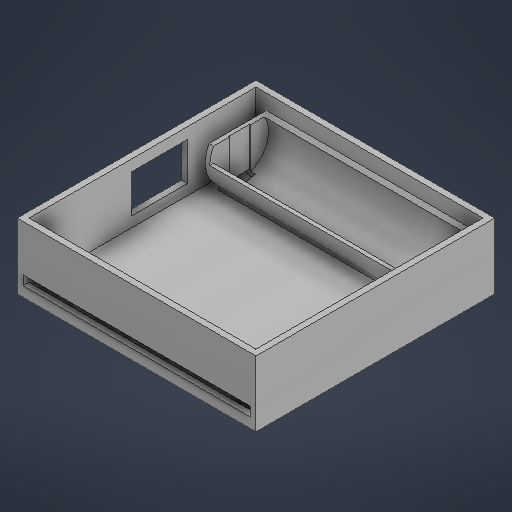
# Autodesk Inventor part: obudowa2
Saved by Autodesk Inventor 2026.1 (Build 301233000, 233)
## iProperties
Created: 2025-08-19
Part Number: obudowa2
Material: Generic
Document SubType Name: Modeling
Designer: Paweł
Density: 1 g/cm^3
Appearance: Light Gray
Mass: 30.7875 g
Surface Area: 279.129 cm^2
Volume: 30.7875 cm^3
Author: Paweł
Autodesk Inventor part; units mm, degrees
ref_plane "YZ Plane" through (0, 0, 0) normal (1, 0, 0) x (0, 1, 0)
ref_plane "XZ Plane" through (0, 0, 0) normal (0, 1, 0) x (-1, 0, 0)
sketch "Sketch1" plane through (0, 0, 0) normal (0, 1, 0) x (-1, 0, 0)
  line L0 (77.0121, 67.7143) -> (-2.9879, 67.7143)
  line L1 (-2.9879, 67.7143) -> (-2.9879, -12.2857)
  line L2 (-2.9879, -12.2857) -> (77.0121, -12.2857)
  line L3 (77.0121, -12.2857) -> (77.0121, 67.7143)
  point P0 (0, 0)
  dimension "d0" = 80
  dimension "d1" = 80
  constraints: 8 end point, 2 parallel, 1 horizontal, 1 perpendicular
  measures "d0" distance of L2.end L1.end
  measures "d1" distance of L0.end L1.end
extrude "Extrusion1" add sketch "Sketch1" along normal blind 2
sketch "Sketch2" plane through (0, 2, 0) normal (0, 1, 0) x (1, 0, 0)
  line L0 (2.9879, -67.7143) -> (2.9879, 12.2857) projected
  line L1 (2.9879, 12.2857) -> (-77.0121, 12.2857) projected
  line L2 (-77.0121, 12.2857) -> (-77.0121, -67.7143) projected
  line L3 (-77.0121, -67.7143) -> (2.9879, -67.7143) projected
  line L4 (0.9879, -65.7143) -> (0.9879, 10.2857)
  line L5 (0.9879, 10.2857) -> (-75.0121, 10.2857)
  line L6 (-75.0121, 10.2857) -> (-75.0121, -65.7143)
  line L7 (-75.0121, -65.7143) -> (0.9879, -65.7143)
  point P0 (0, 0)
  dimension "d4" = 2
  constraints: 8 end point, 3 other
  measures "d4" distance between parallel lines of L3 L7
extrude "Extrusion2" add sketch "Sketch2" along normal blind 20
sketch "Sketch4" plane through (-77.0121, 0, 67.7143) normal (0, 0, 1) x (1, 0, 0)
  line L0 (2, 2) -> (2, 22) projected
  line L1 (78, 2) -> (78, 22) projected
  line L2 (2, 12) -> (78, 12)
  line L3 (78, 12) -> (78, 2)
  line L4 (78, 2) -> (2, 2)
  line L5 (2, 2) -> (2, 12)
  line L6 (2, 2) -> (78, 2)
  line L7 (78, 2) -> (78, 7)
  line L8 (78, 7) -> (2, 7)
  line L9 (2, 7) -> (2, 2)
  line L10 (78, 2) -> (62, 2)
  line L11 (62, 2) -> (2, 2)
  line L12 (2, 2) -> (78, 2) projected
  line L13 (2, 2) -> (62, 2)
  line L14 (2, 3.4) -> (78, 3.4)
  line L15 (2, 6.5) -> (78, 6.5)
  point P0 (77.0121, 0)
  point P1 (2, 3.4)
  dimension "d53" = 16
  dimension "d54" = 1.4
  dimension "d55" = 0.5
  constraints: 26 end point, 5 parallel, 5 point on line, 2 collinear, 2 horizontal, 2 midpoint, 2 perpendicular
  measures "d53" distance of L6.end L10.end
  measures "d54" distance between parallel lines of L4 L14
  measures "d55" distance between parallel lines of L8 L15
extrude "Extrusion4" cut sketch "Sketch4" against normal blind 20 contours L0 L15 L1 L14
sketch "Sketch5" plane through (0.9879, 2, -10.2857) normal (-1, 0, 0) x (0, 0, 1)
  line L0 (76, 0) -> (0, 0) projected
  line L1 (0, 0) -> (0, 20) projected
  circle A0 centre (10, 10) radius 9
  circle A1 centre (10, 10) radius 10
  circle A2 centre (10, 10) radius 10.5
  circle A3 centre (10, 10) radius 9.2
  line L2 (0, 20) -> (76, 20) projected
  line L3 (0, 10) -> (20.5, 10)
  line L4 (13.2016, 0) -> (16.2016, 0)
  line L5 (16.2016, 0) -> (16.2016, 1.5271)
  line L6 (10, 10) -> (10, 20)
  point P0 (10.2857, -2)
  point P1 (78, 0)
  point P2 (10, 0)
  point P3 (13.2016, 0)
  point P4 (13.2016, 20)
  point P5 (6.7984, 20)
  point P6 (0, 13.2016)
  point P7 (0.8, 10)
  point P8 (0, 10)
  point P9 (19.2, 10)
  point P10 (6.7984, 0)
  point P11 (0, 6.7984)
  point P12 (10, 19.2)
  dimension "d11" = 18
  dimension "d12" = 1
  dimension "d13" = 0.5
  dimension "d14" = 0.2
  dimension "d31" = 3
  constraints: 8 end point, 5 point on circle, 4 centre point, 4 midpoint, 4 point on line, 1 horizontal alignment, 1 parallel, 1 perpendicular
  measures "d11" diameter of A0
  measures "d12" radial gap between concentric circles of A0 A1
  measures "d13" radial gap between concentric circles of A1 A2
  measures "d14" radial gap between concentric circles of A0 A3
  measures "d31" distance of L4.start L4.end
extrude "Extrusion5" add sketch "Sketch5" along normal blind 71 contours L0 A2 L5 | L0 A1 L3 A2 | L0 A2 L1 A1 | A1 L3 A3 | L0 L1 A2 | L1 A2 L2 A1 | A1 L6 A3 L3 | L1 L2 A2 picked at (0.4271, 11.4241)
sketch "Sketch10" plane through (0, 2, 0) normal (0, 1, 0) x (1, 0, 0)
  line L0 (-70.0121, -2.9159) -> (-70.0121, -10.2143) projected
  line L1 (-70.0121, 10.2857) -> (-75.0121, 10.2857) projected
  line L2 (-70.0121, -10.2143) -> (-71.5121, -10.2143)
  line L3 (-71.5121, -10.2143) -> (-71.5121, 10.2857)
  line L4 (-71.5121, 10.2857) -> (-70.0121, 10.2857)
  line L5 (-70.0121, 10.2857) -> (-70.0121, -10.2143)
  point P0 (0, 0)
  point P1 (-70.0121, -5.9159)
  dimension "d21" = 1.5
  constraints: 8 end point, 2 parallel, 1 horizontal, 1 perpendicular, 1 point on line
  measures "d21" distance of L3.end L4.end
extrude "Extrusion8" add sketch "Sketch10" along normal up to surface (20 mm away)
sketch "Sketch11" plane through (-71.5121, 2, -10.2857) normal (-1, 0, 0) x (0, 0, 1)
  line L0 (20.5, 0) -> (0, 0) projected
  line L1 (20.5, 0) -> (20.5, 20) projected
  line L2 (0, 0) -> (0, 20) projected
  line L3 (20.5, 0) -> (20.5, 20) projected
  line L4 (0, 15) -> (20.5, 15) projected
  line L5 (6.75, 2) -> (13.75, 2)
  line L6 (13.75, 2) -> (13.75, 0)
  line L7 (0, 0) -> (0, 20) projected
  line L8 (20.5, 0) -> (0, 0) projected
  line L9 (6.75, 2) -> (6.75, 0)
  line L10 (20.5, 20) -> (0, 20) projected
  point P0 (10.2857, -2)
  point P1 (10.25, 2)
  point P2 (10.25, 15)
  dimension "d25" = 2
  dimension "d26" = 7
  constraints: 6 end point, 2 point on line, 1 horizontal, 1 midpoint, 1 parallel, 1 perpendicular, 1 vertical alignment
  measures "d25" distance between parallel lines of L0 L5
  measures "d26" distance of L5.start L5.end
extrude "Extrusion9" cut sketch "Sketch11" along normal blind 4 and the other way blind 3 contours L0 L9 L5 L6
sketch "Sketch14" plane through (-70.0121, 2, 10.2143) normal (1, 0, 0) x (0, 0, -1)
  arc A0 (0, 10) -> (4.2984, 1.5271) centre (10.5, 10) ccw projected
  line L0 (0, 0) -> (0, 10) projected
  line L1 (4.2984, 0) -> (0, 0) projected
  line L2 (4.2984, 0) -> (4.2984, 1.5271) projected
  point P0 (10.2143, -2)
extrude "Extrusion11" cut sketch "Sketch14" against normal up to surface (5 mm away)
sketch "Sketch15" plane through (-70.0121, 12, 10.2143) normal (1, 0, 0) x (0, 0, -1)
  line L0 (4.2984, -10) -> (4.2984, -8.4729) projected
  line L1 (4.2984, -10) -> (4.2984, 5)
  line L2 (13.75, -8) -> (6.75, -8)
  line L3 (6.75, -8) -> (6.75, 5)
  line L4 (6.75, 5) -> (13.75, 5)
  line L5 (13.75, 5) -> (13.75, -8)
  point P0 (10.2143, -12)
  dimension "d35" = 15
  constraints: 10 end point, 2 parallel, 1 horizontal, 1 perpendicular, 1 vertical
  measures "d35" distance of L0.start L1.end
extrude "Extrusion12" cut sketch "Sketch15" against normal blind 0.3
sketch "Sketch16" plane through (-70.0121, 12, 10.2143) normal (1, 0, 0) x (0, 0, -1)
  arc A0 (13.75, -8.6068) -> (10.5, 9.2) centre (10.5, 0) ccw projected
  arc A1 (0, 0) -> (4.2984, -8.4729) centre (10.5, 0) ccw projected
  circle A2 centre (10.5, 0) radius 10.5
  line L0 (10.5, 10) -> (0, 10) projected
  line L1 (0, 0) -> (0, 10) projected
  point P0 (10.2143, -12)
  point P1 (0, 0)
  point P2 (7.2984, 10)
  constraints: 1 centre point, 1 coincident, 1 concentric
extrude "Extrusion13" cut sketch "Sketch16" against normal up to surface (5 mm away) contours L1 L0 A2
sketch "Sketch17" plane through (-77.0121, 0, -12.2857) normal (-1, 0, 0) x (0, 0, 1)
  line L0 (0, 0) -> (0, 22) projected
  line L1 (25.5, 18) -> (43, 18)
  line L2 (43, 18) -> (43, 5.5)
  line L3 (43, 5.5) -> (25.5, 5.5)
  line L4 (25.5, 5.5) -> (25.5, 18)
  line L5 (0, 22) -> (80, 22) projected
  line L6 (43, 18) -> (43.7211, 18)
  line L7 (43.7211, 18) -> (43.7211, 5.5)
  line L8 (43.7211, 5.5) -> (43, 5.5)
  line L9 (25.5, 18) -> (25, 18)
  line L10 (25, 18) -> (25, 5.5)
  line L11 (25, 5.5) -> (25.5, 5.5)
  line L12 (25, 18) -> (25, 18.3)
  line L13 (25, 18.3) -> (43.7211, 18.3)
  line L14 (43.7211, 18.3) -> (43.7211, 18)
  point P0 (12.2857, 0)
  point P1 (20.2416, 9.7558)
  point P2 (0, 11)
  dimension "d46" = 12.5
  dimension "d47" = 17.5
  dimension "d50" = 4
  dimension "d51" = 0.5
  dimension "d52" = 0.3
  constraints: 26 end point, 7 perpendicular, 3 horizontal, 2 parallel, 1 midpoint, 1 vertical
  measures "d46" distance of L1.end L2.end
  measures "d47" distance of L2.end L3.end
  measures "d50" distance between parallel lines of L5 L1
  measures "d51" distance of L1.start L9.end
  measures "d52" distance of L9.end L12.end
extrude "Extrusion14" cut sketch "Sketch17" against normal blind 4
sketch "Sketch18" plane through (0.9879, 6.5, 65.7143) normal (-1, 0, 0) x (0, 0, 1)
  arc A0 (-66, 14.7) -> (-56.8, 5.5) centre (-66, 5.5) ccw projected
  point P0 (-65.7143, -6.5)
ref_plane "Work Plane1" through (0.9879, 12, 10.2143) normal (0, 0, 1) x (1, 0, 0)
sketch "Sketch19" plane through (0.9879, 12, 10.2143) normal (0, 0, 1) x (1, 0, 0)
  line L0 (-71, -8.401) -> (-71, 5) projected
  line L1 (-74.2989, 5) -> (0, 5)
  line L2 (0, 5) -> (0, 10)
  line L3 (0, 10) -> (-74.2989, 10)
  line L4 (-74.2989, 10) -> (-74.2989, 5)
  point P0 (-0.9879, -12)
  constraints: 8 end point, 2 parallel, 1 horizontal, 1 perpendicular
extrude "Extrusion15" cut sketch "Sketch19" against normal up to surface (20.5 mm away)
body "Solid1"
